void16-redux-mod-voronoi (Autodesk Fusion 360 design; units mm, degrees)
Autodesk Fusion 360 part; units mm, degrees
note: some values were not read from the file. Chosen so that the rebuilt part matches the saved one: which bodies a step acts on.
(part 1 of 2)
sketch "Sketch572" plane through (0, 0, 0) normal (0, 0, 1) x (1, 0, 0)
  line L0 (0, -3.5) -> (84.45, -3.5)
  line L1 (84.45, -3.5) -> (84.45, 110.5)
  line L2 (84.45, 110.5) -> (0, 110.5)
  line L3 (0, 110.5) -> (0, -3.5)
extrude "Extrude566" add sketch "Sketch572" along normal blind 28 makes body 1
sketch "Sketch573" plane through (0, 0, 0) normal (0, 0, 1) x (1, 0, 0)
  line L0 (0, -1.5) -> (0, -3.5)
  line L1 (0, -3.5) -> (2, -3.5)
  arc A0 (0, -1.5) -> (2, -3.5) centre (2, -1.5) ccw
  line L2 (82.45, -3.5) -> (84.45, -3.5)
  line L3 (84.45, -3.5) -> (84.45, -1.5)
  arc A1 (82.45, -3.5) -> (84.45, -1.5) centre (82.45, -1.5) ccw
  line L4 (0, 108.5) -> (0, 110.5)
  line L5 (0, 110.5) -> (2, 110.5)
  arc A2 (2, 110.5) -> (0, 108.5) centre (2, 108.5) ccw
  line L6 (84.45, 108.5) -> (84.45, 110.5)
  line L7 (84.45, 110.5) -> (82.45, 110.5)
  arc A3 (84.45, 108.5) -> (82.45, 110.5) centre (82.45, 108.5) ccw
extrude "Extrude567" cut sketch "Sketch573" along normal blind 29 from surface at -0.5 bodies 1
sketch "Sketch574" plane through (0, 0, 0) normal (0, 0, 1) x (1, 0, 0)
  line L0 (2.5, -1) -> (81.95, -1)
  line L1 (81.95, -1) -> (81.95, 108)
  line L2 (81.95, 108) -> (2.5, 108)
  line L3 (2.5, 108) -> (2.5, -1)
extrude "Extrude568" cut sketch "Sketch574" along normal blind 32 from surface at 3 bodies 1
sketch "Sketch575" plane through (0, 0, 0) normal (0, 0, 1) x (1, 0, 0)
  line L0 (0, -3.5) -> (9.5938, -3.5)
  line L1 (9.5938, -3.5) -> (9.1335, 3.9995)
  line L2 (9.1335, 3.9995) -> (0, 8.5442)
  line L3 (0, 8.5442) -> (0, -3.5)
  line L4 (12.0985, -3.5) -> (18.3911, -3.5)
  line L5 (18.3911, -3.5) -> (18.0613, 5.0352)
  line L6 (18.0613, 5.0352) -> (16.3047, 5.9151)
  line L7 (16.3047, 5.9151) -> (11.6393, 3.9832)
  line L8 (11.6393, 3.9832) -> (12.0985, -3.5)
  line L9 (28.2832, -3.5) -> (32.7635, -3.5)
  line L10 (32.7635, -3.5) -> (33.7632, 2.8558)
  line L11 (33.7632, 2.8558) -> (27.7947, 7.4257)
  line L12 (27.7947, 7.4257) -> (26.2488, 6.2436)
  line L13 (26.2488, 6.2436) -> (28.2832, -3.5)
  line L14 (35.2942, -3.5) -> (42.0807, -3.5)
  line L15 (42.0807, -3.5) -> (38.4125, 3.9707)
  line L16 (38.4125, 3.9707) -> (36.2593, 2.6358)
  line L17 (36.2593, 2.6358) -> (35.2942, -3.5)
  line L18 (47.3257, -3.5) -> (55.0973, -3.5)
  line L19 (55.0973, -3.5) -> (54.5198, 3.2184)
  line L20 (54.5198, 3.2184) -> (50.3743, 5.4144)
  line L21 (50.3743, 5.4144) -> (48.1848, 4.5961)
  line L22 (48.1848, 4.5961) -> (47.3257, -3.5)
  line L23 (65.7275, 0.3641) -> (66.0747, 4.2167)
  line L24 (66.0747, 4.2167) -> (62.9422, 6.9148)
  line L25 (62.9422, 6.9148) -> (58.4517, 4.1915)
  line L26 (58.4517, 4.1915) -> (65.7275, 0.3641)
  line L27 (67.9938, -3.5) -> (84.45, -3.5)
  line L28 (84.45, -3.5) -> (84.45, -1.6781)
  line L29 (84.45, -1.6781) -> (73.5187, 5.0876)
  line L30 (73.5187, 5.0876) -> (68.5438, 3.7617)
  line L31 (68.5438, 3.7617) -> (68.0524, -1.6911)
  line L32 (68.0524, -1.6911) -> (67.9938, -3.5)
  line L33 (17.4974, 14.9007) -> (17.5932, 8.0658)
  line L34 (17.5932, 8.0658) -> (19.4771, 7.1222)
  line L35 (19.4771, 7.1222) -> (24.3515, 7.94)
  line L36 (24.3515, 7.94) -> (26.628, 9.6807)
  line L37 (26.628, 9.6807) -> (27.2775, 14.3423)
  line L38 (27.2775, 14.3423) -> (22.9787, 16.94)
  line L39 (22.9787, 16.94) -> (17.4974, 14.9007)
  line L40 (29.7772, 14.1667) -> (29.1338, 9.549)
  line L41 (29.1338, 9.549) -> (35.1883, 4.9133)
  line L42 (35.1883, 4.9133) -> (38.1934, 6.7763)
  line L43 (38.1934, 6.7763) -> (39.7695, 8.0899)
  line L44 (39.7695, 8.0899) -> (38.6804, 13.743)
  line L45 (38.6804, 13.743) -> (33.0704, 15.838)
  line L46 (33.0704, 15.838) -> (29.7772, 14.1667)
  line L47 (41.1504, 14.1374) -> (42.229, 8.5388)
  line L48 (42.229, 8.5388) -> (47.0139, 6.8273)
  line L49 (47.0139, 6.8273) -> (49.3539, 7.7019)
  line L50 (49.3539, 7.7019) -> (50.5571, 14.6378)
  line L51 (50.5571, 14.6378) -> (45.7034, 17.5514)
  line L52 (45.7034, 17.5514) -> (41.1504, 14.1374)
  line L53 (64.1082, 13.4115) -> (64.2958, 9.0485)
  line L54 (64.2958, 9.0485) -> (67.693, 6.1222)
  line L55 (67.693, 6.1222) -> (72.5495, 7.4166)
  line L56 (72.5495, 7.4166) -> (73.0869, 13.5316)
  line L57 (73.0869, 13.5316) -> (68.6367, 15.9672)
  line L58 (68.6367, 15.9672) -> (64.1082, 13.4115)
  line L59 (84.45, 1.262) -> (84.45, 16.7844)
  line L60 (84.45, 16.7844) -> (75.5807, 13.3511)
  line L61 (75.5807, 13.3511) -> (75.0306, 7.092)
  line L62 (75.0306, 7.092) -> (84.45, 1.262)
  line L63 (0, 24.6419) -> (0, 13.7038)
  line L64 (0, 13.7038) -> (10.6487, 19.0743)
  line L65 (10.6487, 19.0743) -> (10.4802, 23.8257)
  line L66 (10.4802, 23.8257) -> (3.3627, 26.8204)
  line L67 (3.3627, 26.8204) -> (0, 24.6419)
  line L68 (12.9711, 24.1247) -> (13.1512, 19.0456)
  line L69 (13.1512, 19.0456) -> (16.3589, 17.1445)
  line L70 (16.3589, 17.1445) -> (21.7934, 19.1664)
  line L71 (21.7934, 19.1664) -> (21.4341, 24.0717)
  line L72 (21.4341, 24.0717) -> (15.5962, 26.4591)
  line L73 (15.5962, 26.4591) -> (12.9711, 24.1247)
  line L74 (23.914, 24.4368) -> (24.308, 19.0577)
  line L75 (24.308, 19.0577) -> (28.6821, 16.4145)
  line L76 (28.6821, 16.4145) -> (31.8341, 18.0142)
  line L77 (31.8341, 18.0142) -> (32.5774, 24.0793)
  line L78 (32.5774, 24.0793) -> (26.9027, 27.276)
  line L79 (26.9027, 27.276) -> (23.914, 24.4368)
  line L80 (35.0947, 24.0681) -> (34.3544, 18.0272)
  line L81 (34.3544, 18.0272) -> (39.5721, 16.0787)
  line L82 (39.5721, 16.0787) -> (44.3657, 19.6731)
  line L83 (44.3657, 19.6731) -> (44.3045, 23.3989)
  line L84 (44.3045, 23.3989) -> (39.1405, 27.0251)
  line L85 (39.1405, 27.0251) -> (35.0947, 24.0681)
  line L86 (46.8046, 23.4107) -> (46.8644, 19.7703)
  line L87 (46.8644, 19.7703) -> (52.0665, 16.6476)
  line L88 (52.0665, 16.6476) -> (56.5667, 18.2936)
  line L89 (56.5667, 18.2936) -> (56.6261, 23.5251)
  line L90 (56.6261, 23.5251) -> (50.9806, 26.3187)
  line L91 (50.9806, 26.3187) -> (46.8046, 23.4107)
  line L92 (59.1283, 23.7061) -> (59.0645, 18.0861)
  line L93 (59.0645, 18.0861) -> (62.8752, 15.5863)
  line L94 (62.8752, 15.5863) -> (67.4847, 18.1878)
  line L95 (67.4847, 18.1878) -> (68.5198, 24.8801)
  line L96 (68.5198, 24.8801) -> (62.8789, 26.8335)
  line L97 (62.8789, 26.8335) -> (59.1283, 23.7061)
  line L98 (84.45, 19.4652) -> (84.45, 21.1436)
  line L99 (84.45, 21.1436) -> (73.5373, 26.3106)
  line L100 (73.5373, 26.3106) -> (71.0566, 24.9259)
  line L101 (71.0566, 24.9259) -> (69.9967, 18.0728)
  line L102 (69.9967, 18.0728) -> (74.4942, 15.6113)
  line L103 (74.4942, 15.6113) -> (84.45, 19.4652)
  line L104 (4.7066, 28.9673) -> (11.4594, 26.1259)
  line L105 (11.4594, 26.1259) -> (14.1071, 28.4805)
  line L106 (14.1071, 28.4805) -> (14.1908, 33.5736)
  line L107 (14.1908, 33.5736) -> (9.2969, 36.221)
  line L108 (9.2969, 36.221) -> (6.0759, 34.5401)
  line L109 (6.0759, 34.5401) -> (4.7066, 28.9673)
  line L110 (16.6907, 33.5503) -> (16.6118, 28.7448)
  line L111 (16.6118, 28.7448) -> (22.3492, 26.3985)
  line L112 (22.3492, 26.3985) -> (25.4548, 29.3487)
  line L113 (25.4548, 29.3487) -> (25.3909, 34.4579)
  line L114 (25.3909, 34.4579) -> (22.5593, 36.6355)
  line L115 (22.5593, 36.6355) -> (16.6907, 33.5503)
  line L116 (27.8953, 34.1174) -> (27.9524, 29.5541)
  line L117 (27.9524, 29.5541) -> (33.8321, 26.2419)
  line L118 (33.8321, 26.2419) -> (37.8625, 29.1876)
  line L119 (37.8625, 29.1876) -> (37.7669, 33.732)
  line L120 (37.7669, 33.732) -> (34.4771, 35.8382)
  line L121 (34.4771, 35.8382) -> (27.8953, 34.1174)
  line L122 (40.2683, 33.6924) -> (40.3623, 29.222)
  line L123 (40.3623, 29.222) -> (45.5468, 25.5813)
  line L124 (45.5468, 25.5813) -> (49.6527, 28.4405)
  line L125 (49.6527, 28.4405) -> (49.9378, 34.5492)
  line L126 (49.9378, 34.5492) -> (45.9679, 36.8072)
  line L127 (45.9679, 36.8072) -> (40.2683, 33.6924)
  line L128 (52.4319, 34.3637) -> (52.1594, 28.5247)
  line L129 (52.1594, 28.5247) -> (57.7096, 25.7783)
  line L130 (57.7096, 25.7783) -> (61.2439, 28.7253)
  line L131 (61.2439, 28.7253) -> (60.3685, 32.9277)
  line L132 (60.3685, 32.9277) -> (55.7232, 35.5484)
  line L133 (55.7232, 35.5484) -> (52.4319, 34.3637)
  line L134 (62.8536, 33.2568) -> (63.6998, 29.1949)
  line L135 (63.6998, 29.1949) -> (69.7944, 27.0844)
  line L136 (69.7944, 27.0844) -> (72.2993, 28.4826)
  line L137 (72.2993, 28.4826) -> (72.7061, 33.4194)
  line L138 (72.7061, 33.4194) -> (67.6468, 37.2404)
  line L139 (67.6468, 37.2404) -> (62.8536, 33.2568)
  line L140 (84.45, 23.9097) -> (84.45, 40.4504)
  line L141 (84.45, 40.4504) -> (75.2087, 33.3483)
  line L142 (75.2087, 33.3483) -> (74.8071, 28.4754)
  line L143 (74.8071, 28.4754) -> (84.45, 23.9097)
  line L144 (2.1055, 41.2203) -> (4.9302, 36.9105)
  line L145 (4.9302, 36.9105) -> (5.0583, 36.829)
  line L146 (5.0583, 36.829) -> (8.1291, 38.4315)
  line L147 (8.1291, 38.4315) -> (8.7625, 44.9281)
  line L148 (8.7625, 44.9281) -> (5.114, 46.9429)
  line L149 (5.114, 46.9429) -> (3.1764, 45.3012)
  line L150 (3.1764, 45.3012) -> (2.1055, 41.2203)
  line L151 (11.2619, 44.8) -> (10.6321, 38.3411)
  line L152 (10.6321, 38.3411) -> (15.4615, 35.7285)
  line L153 (15.4615, 35.7285) -> (21.3912, 38.8458)
  line L154 (21.3912, 38.8458) -> (21.1586, 42.7915)
  line L155 (21.1586, 42.7915) -> (15.9886, 47.0495)
  line L156 (15.9886, 47.0495) -> (11.2619, 44.8)
  line L157 (23.6638, 42.778) -> (23.9007, 38.7577)
  line L158 (23.9007, 38.7577) -> (26.9097, 36.4437)
  line L159 (26.9097, 36.4437) -> (33.4266, 38.1475)
  line L160 (33.4266, 38.1475) -> (33.3406, 44.2394)
  line L161 (33.3406, 44.2394) -> (29.0152, 46.4456)
  line L162 (29.0152, 46.4456) -> (23.6638, 42.778)
  line L163 (35.8399, 44.3097) -> (35.9307, 37.876)
  line L164 (35.9307, 37.876) -> (39.0529, 35.8772)
  line L165 (39.0529, 35.8772) -> (44.7125, 38.9701)
  line L166 (44.7125, 38.9701) -> (44.5965, 43.8915)
  line L167 (44.5965, 43.8915) -> (40.3784, 47.0399)
  line L168 (40.3784, 47.0399) -> (35.8399, 44.3097)
  line L169 (47.0984, 43.8421) -> (47.213, 38.9751)
  line L170 (47.213, 38.9751) -> (51.3401, 36.6277)
  line L171 (51.3401, 36.6277) -> (54.7875, 37.8686)
  line L172 (54.7875, 37.8686) -> (56.2956, 43.9099)
  line L173 (56.2956, 43.9099) -> (51.1457, 46.3401)
  line L174 (51.1457, 46.3401) -> (47.0984, 43.8421)
  line L175 (58.8345, 43.7586) -> (57.282, 37.5394)
  line L176 (57.282, 37.5394) -> (61.3403, 35.2498)
  line L177 (61.3403, 35.2498) -> (66.3216, 39.3897)
  line L178 (66.3216, 39.3897) -> (66.088, 43.0389)
  line L179 (66.088, 43.0389) -> (62.1786, 45.5288)
  line L180 (62.1786, 45.5288) -> (58.8345, 43.7586)
  line L181 (5.9736, 49.3241) -> (10.1288, 47.0295)
  line L182 (10.1288, 47.0295) -> (15.0301, 49.362)
  line L183 (15.0301, 49.362) -> (15.6587, 53.6239)
  line L184 (15.6587, 53.6239) -> (11.3443, 57.7846)
  line L185 (11.3443, 57.7846) -> (4.5323, 53.1976)
  line L186 (4.5323, 53.1976) -> (5.9736, 49.3241)
  line L187 (18.1314, 53.2549) -> (17.5091, 49.0359)
  line L188 (17.5091, 49.0359) -> (22.4432, 44.9723)
  line L189 (22.4432, 44.9723) -> (27.6555, 48.5444)
  line L190 (27.6555, 48.5444) -> (27.5474, 53.0485)
  line L191 (27.5474, 53.0485) -> (21.7746, 55.1009)
  line L192 (21.7746, 55.1009) -> (18.1314, 53.2549)
  line L193 (30.0403, 53.3739) -> (30.1531, 48.6716)
  line L194 (30.1531, 48.6716) -> (34.5299, 46.4392)
  line L195 (34.5299, 46.4392) -> (39.1917, 49.2435)
  line L196 (39.1917, 49.2435) -> (39.1152, 53.9062)
  line L197 (39.1152, 53.9062) -> (33.237, 56.1053)
  line L198 (33.237, 56.1053) -> (30.0403, 53.3739)
  line L199 (41.611, 54.1823) -> (41.6931, 49.1782)
  line L200 (41.6931, 49.1782) -> (45.8985, 46.0393)
  line L201 (45.8985, 46.0393) -> (49.8653, 48.4877)
  line L202 (49.8653, 48.4877) -> (50.2706, 54.1099)
  line L203 (50.2706, 54.1099) -> (45.0819, 56.9347)
  line L204 (45.0819, 56.9347) -> (41.611, 54.1823)
  line L205 (52.765, 53.9424) -> (52.3745, 48.5247)
  line L206 (52.3745, 48.5247) -> (57.7247, 45.9998)
  line L207 (57.7247, 45.9998) -> (60.9835, 47.7249)
  line L208 (60.9835, 47.7249) -> (60.9612, 53.104)
  line L209 (60.9612, 53.104) -> (56.3989, 55.3457)
  line L210 (56.3989, 55.3457) -> (52.765, 53.9424)
  line L211 (63.4607, 53.2407) -> (63.4838, 47.6615)
  line L212 (63.4838, 47.6615) -> (67.3696, 45.1866)
  line L213 (67.3696, 45.1866) -> (73.5414, 48.2671)
  line L214 (73.5414, 48.2671) -> (72.5144, 54.1165)
  line L215 (72.5144, 54.1165) -> (68.4625, 56.7928)
  line L216 (68.4625, 56.7928) -> (63.4607, 53.2407)
  line L217 (84.45, 43.7394) -> (84.45, 58.9147)
  line L218 (84.45, 58.9147) -> (75.0441, 54.1652)
  line L219 (75.0441, 54.1652) -> (76.0615, 48.3703)
  line L220 (76.0615, 48.3703) -> (84.45, 43.7394)
  line L221 (0, 69.0808) -> (0, 56.6662)
  line L222 (0, 56.6662) -> (2.9358, 55.1366)
  line L223 (2.9358, 55.1366) -> (10.1876, 60.0197)
  line L224 (10.1876, 60.0197) -> (9.914, 63.973)
  line L225 (9.914, 63.973) -> (1.8674, 69.0503)
  line L226 (1.8674, 69.0503) -> (0, 69.0808)
  line L227 (12.4205, 63.9653) -> (12.6983, 59.952)
  line L228 (12.6983, 59.952) -> (17.2171, 55.5942)
  line L229 (17.2171, 55.5942) -> (20.5627, 57.2894)
  line L230 (20.5627, 57.2894) -> (21.8412, 64.719)
  line L231 (21.8412, 64.719) -> (16.3821, 66.0508)
  line L232 (16.3821, 66.0508) -> (12.4205, 63.9653)
  line L233 (24.3951, 64.8189) -> (23.0984, 57.2836)
  line L234 (23.0984, 57.2836) -> (28.514, 55.3581)
  line L235 (28.514, 55.3581) -> (31.6396, 58.0287)
  line L236 (31.6396, 58.0287) -> (30.6879, 63.9531)
  line L237 (30.6879, 63.9531) -> (27.2484, 66.233)
  line L238 (27.2484, 66.233) -> (24.3951, 64.8189)
  line L239 (33.2272, 63.9078) -> (34.104, 58.4502)
  line L240 (34.104, 58.4502) -> (40.1276, 56.1966)
  line L241 (40.1276, 56.1966) -> (43.7319, 59.0548)
  line L242 (43.7319, 59.0548) -> (43.9492, 63.5829)
  line L243 (43.9492, 63.5829) -> (39.4165, 66.4165)
  line L244 (39.4165, 66.4165) -> (33.2272, 63.9078)
  line L245 (46.452, 63.5807) -> (46.2394, 59.1511)
  line L246 (46.2394, 59.1511) -> (51.6647, 56.1974)
  line L247 (51.6647, 56.1974) -> (55.2211, 57.5708)
  line L248 (55.2211, 57.5708) -> (55.3137, 64.1101)
  line L249 (55.3137, 64.1101) -> (49.9567, 66.0238)
  line L250 (49.9567, 66.0238) -> (46.452, 63.5807)
  line L251 (57.8158, 64.2432) -> (57.7201, 57.482)
  line L252 (57.7201, 57.482) -> (62.0912, 55.3343)
  line L253 (62.0912, 55.3343) -> (67.1656, 58.9382)
  line L254 (67.1656, 58.9382) -> (67.0042, 63.8929)
  line L255 (67.0042, 63.8929) -> (62.2691, 66.7036)
  line L256 (62.2691, 66.7036) -> (57.8158, 64.2432)
  line L257 (84.45, 61.7153) -> (84.45, 63.8136)
  line L258 (84.45, 63.8136) -> (77.4052, 69.187)
  line L259 (77.4052, 69.187) -> (69.5033, 63.9609)
  line L260 (69.5033, 63.9609) -> (69.6651, 58.9946)
  line L261 (69.6651, 58.9946) -> (73.7363, 56.3055)
  line L262 (73.7363, 56.3055) -> (84.45, 61.7153)
  line L263 (4.2762, 70.4864) -> (11.1737, 66.1342)
  line L264 (11.1737, 66.1342) -> (15.008, 68.1527)
  line L265 (15.008, 68.1527) -> (15.4108, 75.727)
  line L266 (15.4108, 75.727) -> (11.9553, 77.6511)
  line L267 (11.9553, 77.6511) -> (4.2762, 70.4864)
  line L268 (17.9008, 75.4729) -> (17.5218, 68.3461)
  line L269 (17.5218, 68.3461) -> (23.1243, 66.9793)
  line L270 (23.1243, 66.9793) -> (26.1217, 68.4648)
  line L271 (26.1217, 68.4648) -> (26.3453, 73.6548)
  line L272 (26.3453, 73.6548) -> (22.046, 76.6112)
  line L273 (22.046, 76.6112) -> (17.9008, 75.4729)
  line L274 (28.8457, 73.6109) -> (28.6179, 68.3246)
  line L275 (28.6179, 68.3246) -> (31.9764, 66.0984)
  line L276 (31.9764, 66.0984) -> (38.2604, 68.6454)
  line L277 (38.2604, 68.6454) -> (38.0989, 73.5822)
  line L278 (38.0989, 73.5822) -> (33.2869, 76.6232)
  line L279 (33.2869, 76.6232) -> (28.8457, 73.6109)
  line L280 (40.6009, 73.5622) -> (40.7658, 68.5213)
  line L281 (40.7658, 68.5213) -> (45.1954, 65.7522)
  line L282 (45.1954, 65.7522) -> (48.5589, 68.0969)
  line L283 (48.5589, 68.0969) -> (48.9328, 74.3327)
  line L284 (48.9328, 74.3327) -> (46.0081, 76.5598)
  line L285 (46.0081, 76.5598) -> (40.6009, 73.5622)
  line L286 (51.4188, 74.0232) -> (51.0743, 68.2793)
  line L287 (51.0743, 68.2793) -> (56.4655, 66.3533)
  line L288 (56.4655, 66.3533) -> (60.9407, 68.8258)
  line L289 (60.9407, 68.8258) -> (60.267, 73.9347)
  line L290 (60.267, 73.9347) -> (57.3848, 76.1484)
  line L291 (57.3848, 76.1484) -> (51.4188, 74.0232)
  line L292 (67.6869, 76.6064) -> (62.7898, 73.9255)
  line L293 (62.7898, 73.9255) -> (63.4514, 68.9091)
  line L294 (63.4514, 68.9091) -> (68.1953, 66.0931)
  line L295 (68.1953, 66.0931) -> (76.1164, 71.3319)
  line L296 (76.1164, 71.3319) -> (76.0166, 72.0979)
  line L297 (76.0166, 72.0979) -> (67.6869, 76.6064)
  line L298 (0, 83.0517) -> (0, 71.5812)
  line L299 (0, 71.5812) -> (1.7542, 71.5525)
  line L300 (1.7542, 71.5525) -> (10.4214, 79.6391)
  line L301 (10.4214, 79.6391) -> (9.7366, 83.6036)
  line L302 (9.7366, 83.6036) -> (0, 83.0517)
  line L303 (24.0822, 85.0868) -> (23.5774, 78.5921)
  line L304 (23.5774, 78.5921) -> (27.6288, 75.8063)
  line L305 (27.6288, 75.8063) -> (32.0923, 78.8337)
  line L306 (32.0923, 78.8337) -> (32.5475, 82.4904)
  line L307 (32.5475, 82.4904) -> (27.2658, 86.2587)
  line L308 (27.2658, 86.2587) -> (24.0822, 85.0868)
  line L309 (35.0515, 82.3674) -> (34.6012, 78.75)
  line L310 (34.6012, 78.75) -> (39.3682, 75.7373)
  line L311 (39.3682, 75.7373) -> (44.7879, 78.7418)
  line L312 (44.7879, 78.7418) -> (44.2103, 84.3411)
  line L313 (44.2103, 84.3411) -> (40.62, 86.2398)
  line L314 (40.62, 86.2398) -> (35.0515, 82.3674)
  line L315 (46.719, 84.3856) -> (47.3038, 78.7154)
  line L316 (47.3038, 78.7154) -> (50.439, 76.3281)
  line L317 (50.439, 76.3281) -> (56.3587, 78.4368)
  line L318 (56.3587, 78.4368) -> (56.3723, 83.8601)
  line L319 (56.3723, 83.8601) -> (50.2849, 86.089)
  line L320 (50.2849, 86.089) -> (46.719, 84.3856)
  line L321 (58.8729, 84.1362) -> (58.858, 78.1692)
  line L322 (58.858, 78.1692) -> (61.5535, 76.0988)
  line L323 (61.5535, 76.0988) -> (66.4865, 78.7994)
  line L324 (66.4865, 78.7994) -> (66.9203, 84.7231)
  line L325 (66.9203, 84.7231) -> (61.692, 86.424)
  line L326 (61.692, 86.424) -> (58.8729, 84.1362)
  line L327 (72.5997, 86.3423) -> (69.4326, 84.7999)
  line L328 (69.4326, 84.7999) -> (68.9892, 78.7442)
  line L329 (68.9892, 78.7442) -> (76.5476, 74.6532)
  line L330 (76.5476, 74.6532) -> (78.9962, 80.5865)
  line L331 (78.9962, 80.5865) -> (72.5997, 86.3423)
  line L332 (11.1555, 87.0697) -> (15.0434, 90.3681)
  line L333 (15.0434, 90.3681) -> (15.1256, 94.124)
  line L334 (15.1256, 94.124) -> (10.5379, 97.1905)
  line L335 (10.5379, 97.1905) -> (5.4734, 94.7053)
  line L336 (5.4734, 94.7053) -> (11.1555, 87.0697)
  line L337 (31.4995, 98.4229) -> (28.8774, 88.1799)
  line L338 (28.8774, 88.1799) -> (33.8892, 84.6042)
  line L339 (33.8892, 84.6042) -> (39.1354, 88.2525)
  line L340 (39.1354, 88.2525) -> (37.0101, 98.2076)
  line L341 (37.0101, 98.2076) -> (31.6021, 98.4443)
  line L342 (31.6021, 98.4443) -> (31.4995, 98.4229)
  line L343 (39.4217, 98.8856) -> (41.6319, 88.5327)
  line L344 (41.6319, 88.5327) -> (45.4137, 86.5327)
  line L345 (45.4137, 86.5327) -> (49.0932, 88.2904)
  line L346 (49.0932, 88.2904) -> (50.0863, 94.3257)
  line L347 (50.0863, 94.3257) -> (39.6425, 99.048)
  line L348 (39.6425, 99.048) -> (39.4217, 98.8856)
  line L349 (52.6124, 94.2799) -> (51.6221, 88.2617)
  line L350 (51.6221, 88.2617) -> (57.3878, 86.1506)
  line L351 (57.3878, 86.1506) -> (60.1357, 88.3807)
  line L352 (60.1357, 88.3807) -> (59.6428, 94.8014)
  line L353 (59.6428, 94.8014) -> (57.1386, 96.8701)
  line L354 (57.1386, 96.8701) -> (52.6124, 94.2799)
  line L355 (62.1726, 94.5094) -> (62.6145, 88.7529)
  line L356 (62.6145, 88.7529) -> (68.1451, 86.9536)
  line L357 (68.1451, 86.9536) -> (71.7234, 88.6962)
  line L358 (71.7234, 88.6962) -> (72.7403, 93.178)
  line L359 (72.7403, 93.178) -> (68.5318, 96.3546)
  line L360 (68.5318, 96.3546) -> (62.1726, 94.5094)
  line L361 (84.45, 88.1142) -> (84.45, 98.4831)
  line L362 (84.45, 98.4831) -> (76.4474, 93.6273)
  line L363 (76.4474, 93.6273) -> (84.45, 88.1142)
  line L364 (8.2463, 110.5) -> (0, 110.5)
  line L365 (0, 110.5) -> (0, 96.5387)
  line L366 (0, 96.5387) -> (3.3033, 96.4252)
  line L367 (3.3033, 96.4252) -> (9.3074, 99.3715)
  line L368 (9.3074, 99.3715) -> (8.2463, 110.5)
  line L369 (14.1848, 110.5) -> (10.7576, 110.5)
  line L370 (10.7576, 110.5) -> (11.8218, 99.3394)
  line L371 (11.8218, 99.3394) -> (16.3415, 96.3183)
  line L372 (16.3415, 96.3183) -> (16.7779, 96.6519)
  line L373 (16.7779, 96.6519) -> (16.4734, 107.8826)
  line L374 (16.4734, 107.8826) -> (14.1848, 110.5)
  line L375 (54.5213, 110.5) -> (46.5468, 110.5)
  line L376 (46.5468, 110.5) -> (41.2486, 101.0655)
  line L377 (41.2486, 101.0655) -> (51.4088, 96.4715)
  line L378 (51.4088, 96.4715) -> (55.961, 99.0767)
  line L379 (55.961, 99.0767) -> (55.8021, 101.1391)
  line L380 (55.8021, 101.1391) -> (54.5213, 110.5)
  line L381 (58.3855, 100.1523) -> (58.4736, 99.01)
  line L382 (58.4736, 99.01) -> (61.135, 96.8114)
  line L383 (61.135, 96.8114) -> (67.5752, 98.6801)
  line L384 (67.5752, 98.6801) -> (67.6807, 101.1012)
  line L385 (67.6807, 101.1012) -> (58.3855, 100.1523)
extrude "Extrude569" add sketch "Sketch575" along normal blind 36 from surface at -6 separate body makes body 2 at (44.6353, 99.5341, 6) makes body 3 at (0, 105.8462, 6) makes body 4 at (66.4121, 95.7395, 6) makes body 5 at (46.605, 95.8998, 6) makes body 6 at (7.3674, 92.1601, 6) makes body 7 at (58.868, 82.1472, 6) makes body 8 at (38.7639, 84.949, 18) makes body 9 at (4.6433, 74.248, 6) makes body 10 at (55.3961, 75.44, 6) makes body 11 at (36.1657, 67.7964, 18) makes body 12 at (9.3956, 75.2629, 18) makes body 13 at (57.7839, 61.9895, 18) makes body 14 at (37.3534, 65.5803, 6) makes body 15 at (20.9888, 59.766, 18) makes body 16 at (84.45, 48.7978, 6) makes body 17 at (54.1579, 47.6831, 6) makes body 18 at (37.1558, 54.6392, 6) makes body 19 at (19.1538, 47.6814, 6) makes body 20 at (63.0007, 36.6298, 6) makes body 21 at (40.9394, 36.9081, 6) makes body 22 at (17.438, 36.7676, 6) makes body 23 at (84.45, 29.4232, 6) makes body 24 at (54.0095, 27.6092, 6) makes body 25 at (32.2832, 35.2646, 18) makes body 26 at (6.9575, 28.0202, 6) makes body 27 at (67.8298, 20.4186, 6) makes body 28 at (42.5831, 24.6076, 6) makes body 29 at (19.4881, 24.8675, 6) makes body 30 at (84.45, 6.4361, 6) makes body 31 at (49.7549, 10.0139, 18) makes body 32 at (17.5294, 12.6224, 18) makes body 33 at (60.877, 2.9157, 6) makes body 34 at (40.858, -1.0098, 6) makes body 35 at (18.2812, -0.6549, 6) makes body 36 at (26.9269, 2.9957, 6) makes body 37 at (47.8984, 1.8974, 18) makes body 38 at (73.4792, -3.5, 6) makes body 39 at (31.152, 8.0038, 6) makes body 40 at (72.7286, 9.4549, 18) makes body 41 at (3.5496, 15.494, 6) makes body 42 at (30.6858, 25.1449, 6) makes body 43 at (54.7442, 24.4563, 6) makes body 44 at (80.8124, 22.8659, 6) makes body 45 at (20.6031, 35.6071, 6) makes body 46 at (44.068, 35.7689, 6) makes body 47 at (65.7313, 28.4914, 6) makes body 48 at (8.3402, 40.597, 6) makes body 49 at (29.082, 37.0116, 18) makes body 50 at (55.2902, 39.8824, 6) makes body 51 at (9.0737, 56.2556, 6) makes body 52 at (0, 4.5295, 6) makes body 53 at (48.541, 55.0515, 18) makes body 54 at (69.4269, 46.2134, 18) makes body 55 at (0, 64.9426, 6) makes body 56 at (23.9629, 62.3071, 6) makes body 57 at (55.252, 59.7506, 6) makes body 58 at (77.3075, 58.1088, 18) makes body 59 at (17.7745, 73.0973, 6) makes body 60 at (48.6836, 70.1755, 6) makes body 61 at (70.8357, 67.8394, 6) makes body 62 at (23.9139, 82.9219, 6) makes body 63 at (54.3431, 84.6031, 6) makes body 64 at (76.864, 82.5051, 18) makes body 65 at (30.6254, 95.0086, 6) makes body 66 at (59.9714, 90.5209, 6) makes body 67 at (84.45, 91.5705, 6) makes body 68 at (16.6764, 100.3955, 6) makes body 69 at (64.5823, 100.7849, 18)
move_body "Move584" bodies 2 to x (0.991592, 0.008841, 0.129102) y (0.008841, 0.990703, -0.135753) z (-0.129102, 0.135753, 0.982295) at (1.043, -1.0967, 7.986)
move_body "Move585" bodies 3 to x (0.995047, 0.007992, -0.099087) y (0.007992, 0.987106, 0.159865) z (0.099087, -0.159865, 0.982153) at (-1.9928, 3.2152, -15.8648)
move_body "Move586" bodies 4 to x (0.994433, 0.011641, 0.104726) y (0.011641, 0.975656, -0.218996) z (-0.104726, 0.218996, 0.970089) at (0.5653, -1.182, 13.3664)
move_body "Move587" bodies 5 to x (0.988041, -0.017698, -0.153174) y (-0.017698, 0.97381, -0.226673) z (0.153174, 0.226673, 0.961851) at (0.3393, 0.5021, 28.346)
move_body "Move588" bodies 6 to x (0.968969, 0.002343, 0.247172) y (0.002343, 0.999823, -0.018664) z (-0.247172, 0.018664, 0.968792) at (3.0698, -0.2318, -0.4517)
move_body "Move589" bodies 7 to x (0.977564, 0.020464, -0.209644) y (0.020464, 0.981335, 0.191215) z (0.209644, -0.191215, 0.958898) at (-2.7677, 2.5244, -1.8608)
move_body "Move590" bodies 8 to x (0.998968, -0.005949, -0.045022) y (-0.005949, 0.965695, -0.25961) z (0.045022, 0.25961, 0.964663) at (-0.0175, -0.1009, 23.2366)
move_body "Move591" bodies 9 to x (0.987423, 0.004942, 0.158025) y (0.004942, 0.998058, -0.062096) z (-0.158025, 0.062096, 0.985481) at (1.5784, -0.6202, 4.1681)
move_body "Move592" bodies 10 to x (0.99475, -0.01008, -0.101838) y (-0.01008, 0.980646, -0.195532) z (0.101838, 0.195532, 0.975395) at (-0.2098, -0.4028, 19.9308)
move_body "Move593" bodies 11 to x (0.966183, 0.017671, -0.257253) y (0.017671, 0.990766, 0.134424) z (0.257253, -0.134424, 0.956949) at (-3.2172, 1.6811, -0.4737)
move_body "Move594" bodies 12 to x (0.993128, -0.009793, -0.116619) y (-0.009793, 0.986043, -0.166201) z (0.116619, 0.166201, 0.979172) at (-0.6277, -0.8946, 13.3465)
move_body "Move595" bodies 13 to x (0.983187, 0.000142, 0.182601) y (0.000142, 0.999999, -0.001542) z (-0.182601, 0.001542, 0.983186) at (3.2324, -0.0273, -11.1063)
move_body "Move596" bodies 14 to x (0.995747, -0.007957, 0.091783) y (-0.007957, 0.985112, 0.171731) z (-0.091783, -0.171731, 0.980859) at (1.7533, 3.2806, -13.8403)
move_body "Move597" bodies 15 to x (0.994867, -0.009808, 0.100713) y (-0.009808, 0.981258, 0.192447) z (-0.100713, -0.192447, 0.976126) at (1.893, 3.6173, -13.1439)
move_body "Move598" bodies 16 to x (0.9987, 0.003972, 0.050813) y (0.003972, 0.987858, -0.155306) z (-0.050813, 0.155306, 0.986559) at (0.5095, -1.5573, 4.0805)
move_body "Move599" bodies 17 to x (0.968799, -0.018725, 0.247139) y (-0.018725, 0.988762, 0.148319) z (-0.247139, -0.148319, 0.957561) at (5.6829, 3.4106, -21.0141)
move_body "Move600" bodies 18 to x (0.989264, -0.007666, -0.145936) y (-0.007666, 0.994525, -0.104213) z (0.145936, 0.104213, 0.98379) at (-0.9865, -0.7045, 10.5895)
move_body "Move601" bodies 19 to x (0.978538, 0.004975, 0.206004) y (0.004975, 0.998847, -0.047753) z (-0.206004, 0.047753, 0.977385) at (2.7078, -0.6277, -1.9913)
move_body "Move602" bodies 20 to x (0.979527, -0.021522, 0.200161) y (-0.021522, 0.977376, 0.210412) z (-0.200161, -0.210412, 0.956902) at (4.5365, 4.7688, -20.3515)
move_body "Move603" bodies 21 to x (0.976858, -0.005031, -0.213831) y (-0.005031, 0.998906, -0.046487) z (0.213831, 0.046487, 0.975764) at (-1.4253, -0.3099, 10.8304)
move_body "Move604" bodies 22 to x (0.996945, -0.011117, 0.07731) y (-0.011117, 0.959546, 0.281331) z (-0.07731, -0.281331, 0.956491) at (1.4367, 5.2283, -12.3598)
move_body "Move605" bodies 23 to x (0.984696, 0.003078, -0.174254) y (0.003078, 0.999381, 0.03505) z (0.174254, -0.03505, 0.984077) at (-0.9715, 0.1954, 12.9387)
move_body "Move606" bodies 24 to x (0.998925, -0.005398, 0.046044) y (-0.005398, 0.972899, 0.231169) z (-0.046044, -0.231169, 0.971824) at (0.779, 3.9111, -9.361)
move_body "Move607" bodies 25 to x (0.98641, 0.000173, 0.1643) y (0.000173, 0.999998, -0.00209) z (-0.1643, 0.00209, 0.986408) at (2.413, -0.0307, -5.174)
move_body "Move608" bodies 26 to x (0.999988, 0.000678, -0.004883) y (0.000678, 0.962127, 0.272602) z (0.004883, -0.272602, 0.962115) at (-0.0796, 4.4455, -7.9972)
move_body "Move609" bodies 27 to x (0.99916, -0.003341, -0.040854) y (-0.003341, 0.986717, -0.162413) z (0.040854, 0.162413, 0.985877) at (-0.3658, -1.4541, 6.2204)
move_body "Move610" bodies 28 to x (0.990065, 0.014611, -0.139846) y (0.014611, 0.97851, 0.20568) z (0.139846, -0.20568, 0.968576) at (-1.602, 2.3562, 1.4487)
move_body "Move611" bodies 29 to x (0.981598, 0.019624, 0.189947) y (0.019624, 0.979073, -0.202562) z (-0.189947, 0.202562, 0.960671) at (2.1714, -2.3156, 1.5865)
move_body "Move612" bodies 30 to x (0.990758, 0.013688, -0.134949) y (0.013688, 0.979727, 0.199868) z (0.134949, -0.199868, 0.970485) at (-1.0059, 1.4899, 9.3116)
move_body "Move613" bodies 31 to x (0.993364, 0.011438, 0.114445) y (0.011438, 0.980286, -0.197253) z (-0.114445, 0.197253, 0.97365) at (1.5382, -2.6512, -2.5271)
move_body "Move614" bodies 32 to x (0.969777, 0.008933, 0.243828) y (0.008933, 0.997359, -0.072071) z (-0.243828, 0.072071, 0.967137) at (3.4951, -1.0331, -4.1972)
move_body "Move615" bodies 33 to x (0.988391, -0.01512, 0.151179) y (-0.01512, 0.980307, 0.196899) z (-0.151179, -0.196899, 0.968698) at (2.592, 3.3759, -9.7539)
move_body "Move616" bodies 34 to x (0.971429, -0.012616, 0.236996) y (-0.012616, 0.99443, 0.104645) z (-0.236996, -0.104645, 0.965858) at (3.9523, 1.7451, -8.7837)
move_body "Move617" bodies 35 to x (0.997071, -0.010919, -0.075703) y (-0.010919, 0.959297, -0.282187) z (0.075703, 0.282187, 0.956368) at (-0.8513, -3.1731, 2.001)
move_body "Move618" bodies 36 to x (0.996566, 0.006927, 0.082518) y (0.006927, 0.98603, -0.166422) z (-0.082518, 0.166422, 0.982596) at (1.0797, -2.1775, -1.9405)
move_body "Move619" bodies 37 to x (0.99354, -0.01449, 0.112549) y (-0.01449, 0.967495, 0.252474) z (-0.112549, -0.252474, 0.961036) at (1.6953, 3.8029, -5.5379)
move_body "Move620" bodies 38 to x (0.991452, -0.007979, -0.130227) y (-0.007979, 0.992551, -0.121565) z (0.130227, 0.121565, 0.984003) at (-0.9049, -0.8447, 10.2146)
move_body "Move621" bodies 39 to x (0.973167, 0.008063, 0.229958) y (0.008063, 0.997577, -0.069103) z (-0.229958, 0.069103, 0.970744) at (3.6003, -1.0819, -6.8544)
move_body "Move622" bodies 40 to x (0.991536, 0.005832, 0.129704) y (0.005832, 0.995981, -0.089372) z (-0.129704, 0.089372, 0.987517) at (2.0727, -1.4282, -7.7605)
move_body "Move623" bodies 41 to x (0.971876, -0.009017, -0.235321) y (-0.009017, 0.997109, -0.075446) z (0.235321, 0.075446, 0.968985) at (-2.4914, -0.7988, 3.1538)
move_body "Move624" bodies 42 to x (0.991648, 0.00743, 0.128759) y (0.00743, 0.993391, -0.11454) z (-0.128759, 0.11454, 0.985039) at (1.6187, -1.44, -0.9552)
move_body "Move625" bodies 43 to x (0.997956, 0.005882, 0.063632) y (0.005882, 0.983071, -0.183131) z (-0.063632, 0.183131, 0.981027) at (0.7429, -2.1381, 0.8712)
move_body "Move626" bodies 44 to x (0.983544, 0.003396, 0.180639) y (0.003396, 0.999299, -0.037276) z (-0.180639, 0.037276, 0.982843) at (3.3673, -0.6949, -12.9623)
move_body "Move627" bodies 45 to x (0.974924, -0.002209, -0.222529) y (-0.002209, 0.999805, -0.019603) z (0.222529, 0.019603, 0.974729) at (-2.0733, -0.1826, 5.6016)
move_body "Move628" bodies 46 to x (0.990236, -0.006735, -0.139238) y (-0.006735, 0.995354, -0.096044) z (0.139238, 0.096044, 0.98559) at (-1.0204, -0.7038, 9.449)
move_body "Move629" bodies 47 to x (0.987956, -0.002038, -0.154724) y (-0.002038, 0.999655, -0.026183) z (0.154724, 0.026183, 0.987611) at (-0.9748, -0.165, 11.4779)
move_body "Move630" bodies 48 to x (0.989236, 0.009238, 0.146034) y (0.009238, 0.992071, -0.12534) z (-0.146034, 0.12534, 0.981307) at (1.4239, -1.2222, 4.6807)
move_body "Move631" bodies 49 to x (0.997617, 0.007078, -0.068626) y (0.007078, 0.978974, 0.203861) z (0.068626, -0.203861, 0.976592) at (-1.0488, 3.1157, -6.2091)
move_body "Move632" bodies 50 to x (0.991903, 0.015832, -0.126008) y (0.015832, 0.969046, 0.246371) z (0.126008, -0.246371, 0.960949) at (-1.7503, 3.4221, -3.2376)
move_body "Move633" bodies 51 to x (0.99703, 0.010082, 0.076348) y (0.010082, 0.965771, -0.2592) z (-0.076348, 0.2592, 0.962801) at (0.4178, -1.4183, 13.2595)
move_body "Move634" bodies 52 to x (0.990192, 0.007307, 0.139521) y (0.007307, 0.994556, -0.103944) z (-0.139521, 0.103944, 0.984748) at (1.7029, -1.2686, -0.2241)
move_body "Move635" bodies 53 to x (0.987427, -0.017075, 0.157152) y (-0.017075, 0.976812, 0.213416) z (-0.157152, -0.213416, 0.964239) at (3.3426, 4.5393, -17.7787)
move_body "Move636" bodies 54 to x (0.993903, -0.008274, -0.109947) y (-0.008274, 0.988773, -0.149199) z (0.109947, 0.149199, 0.982676) at (-0.4798, -0.6511, 15.347)
move_body "Move637" bodies 55 to x (0.987258, 0.016905, -0.158225) y (0.016905, 0.977571, 0.209928) z (0.158225, -0.209928, 0.964829) at (-2.8838, 3.8261, -11.8104)
move_body "Move638" bodies 56 to x (0.990899, -0.013645, 0.133917) y (-0.013645, 0.979544, 0.200769) z (-0.133917, -0.200769, 0.970442) at (2.6857, 4.0263, -15.5164)
move_body "Move639" bodies 57 to x (0.993027, -0.014789, 0.116952) y (-0.014789, 0.968633, 0.248054) z (-0.116952, -0.248054, 0.961661) at (2.6612, 5.6444, -20.6371)
move_body "Move640" bodies 58 to x (0.966428, -0.013481, -0.256585) y (-0.013481, 0.994587, -0.103031) z (0.256585, 0.103031, 0.961014) at (0.3511, 0.141, 26.6837)
move_body "Move641" bodies 59 to x (0.97952, 0.001733, 0.201341) y (0.001733, 0.999853, -0.017037) z (-0.201341, 0.017037, 0.979373) at (2.7409, -0.2319, -2.9454)
move_body "Move642" bodies 60 to x (0.965663, -0.011692, 0.259535) y (-0.011692, 0.996019, 0.088376) z (-0.259535, -0.088376, 0.961681) at (5.4836, 1.8673, -17.4472)
move_body "Move643" bodies 61 to x (0.964956, -0.003714, 0.262387) y (-0.003714, 0.999606, 0.02781) z (-0.262387, -0.02781, 0.964562) at (5.8476, 0.6198, -19.7825)
move_body "Move644" bodies 62 to x (0.980267, -0.019043, -0.196759) y (-0.019043, 0.981624, -0.189875) z (0.196759, 0.189875, 0.961891) at (-0.2643, -0.255, 21.3649)
move_body "Move645" bodies 63 to x (0.979629, -0.009057, -0.200611) y (-0.009057, 0.995973, -0.089197) z (0.200611, 0.089197, 0.975602) at (-0.6218, -0.2765, 17.8769)
move_body "Move646" bodies 64 to x (0.983624, -0.004796, -0.180169) y (-0.004796, 0.998595, -0.052768) z (0.180169, 0.052768, 0.982219) at (-0.5642, -0.1653, 17.7923)
move_body "Move647" bodies 65 to x (0.981994, 0.006723, -0.188795) y (0.006723, 0.99749, 0.070487) z (0.188795, -0.070487, 0.979484) at (-2.2685, 0.847, 0.2151)
move_body "Move648" bodies 66 to x (0.999183, -0.003871, 0.040235) y (-0.003871, 0.98166, 0.190599) z (-0.040235, -0.190599, 0.980843) at (0.8828, 4.1818, -19.4602)
move_body "Move649" bodies 67 to x (0.985086, -0.020441, -0.170845) y (-0.020441, 0.971985, -0.234152) z (0.170845, 0.234152, 0.957071) at (1.0568, 1.4483, 36.1055)
move_body "Move650" bodies 68 to x (0.997923, -0.005172, 0.064202) y (-0.005172, 0.987118, 0.159913) z (-0.064202, -0.159913, 0.985041) at (1.3339, 3.3223, -17.2409)
move_body "Move651" bodies 69 to x (0.965762, 0.016489, 0.258904) y (0.016489, 0.992059, -0.124689) z (-0.258904, 0.124689, 0.957821) at (3.6333, -1.7498, -3.4746)
combine "Combine170" operation cut target body 1 tool bodies 2 3 4 5 6 7 8 9 10 11 12 13 14 15 16 17 18 19 20 21 22 23 24 25 26 27 28 29 30 31 32 33 34 35 36 37 38 39 40 41 42 43 44 45 46 47 48 49 50 51 52 53 54 55 56 57 58 59 60 61 62 63 64 65 66 67 68 69
sketch "Sketch576" plane through (0, 0, 0) normal (0, 0, 1) x (1, 0, 0)
  circle A0 centre (20, 102.4) radius 3.5
  circle A1 centre (64, 102.4) radius 3.5
  circle A2 centre (4.5, 89) radius 3.5
  circle A3 centre (79.95, 89) radius 3.5
extrude "Extrude570" add sketch "Sketch576" along normal blind 30 separate body makes body 70 at (7.7252, 87.6405, 20) makes body 71 at (67.0738, 100.7261, 20) makes body 72 at (23.0738, 104.0739, 20) makes body 73 at (78.8353, 85.6823, 10)
combine "Combine171" operation add target body 1 tool bodies 70 71 72 73
sketch "Sketch577" plane through (0, 0, 0) normal (0, 0, 1) x (1, 0, 0)
  circle A0 centre (23.175, 0.9) radius 3.25
  circle A1 centre (42.225, 0.9) radius 3.25
  circle A2 centre (61.275, 0.9) radius 3.25
extrude "Extrude571" add sketch "Sketch577" along normal blind 30 separate body makes body 74 at (26.4089, 0.5764, 20) makes body 75 at (45.4589, 0.5764, 20) makes body 76 at (64.5089, 0.5764, 20)
combine "Combine172" operation add target body 1 tool bodies 74 75 76
sketch "Sketch578" plane through (0, 0, 0) normal (0, 0, 1) x (1, 0, 0)
  line L0 (19, 67.7) -> (21, 67.7)
  line L1 (21, 67.7) -> (21, 108.5)
  line L2 (21, 108.5) -> (19, 108.5)
  line L3 (19, 108.5) -> (19, 67.7)
  line L4 (39, 67.7) -> (41, 67.7)
  line L5 (41, 67.7) -> (41, 108.5)
  line L6 (41, 108.5) -> (39, 108.5)
  line L7 (39, 108.5) -> (39, 67.7)
extrude "Extrude572" add sketch "Sketch578" along normal blind 4.5 separate body makes body 77 at (19, 94.9, 1.5) makes body 78 at (39, 94.9, 1.5)
combine "Combine173" operation add target body 1 tool bodies 77 78
sketch "Sketch579" plane through (0, 0, 0) normal (0, 0, 1) x (1, 0, 0)
  line L0 (21, 67.7) -> (39, 67.7)
  line L1 (39, 67.7) -> (39, 108.5)
  line L2 (39, 108.5) -> (21, 108.5)
  line L3 (21, 108.5) -> (21, 67.7)
extrude "Extrude573" add sketch "Sketch579" along normal blind 4.5 separate body makes body 79
combine "Combine174" operation add target body 1 tool bodies 79
sketch "Sketch580" plane through (0, 0, 0) normal (0, 0, 1) x (1, 0, 0)
  line L0 (19, 67.7) -> (21, 67.7)
  line L1 (21, 67.7) -> (21, 108.5)
  line L2 (21, 108.5) -> (19, 108.5)
  line L3 (19, 108.5) -> (19, 67.7)
  line L4 (39, 67.7) -> (41, 67.7)
  line L5 (41, 67.7) -> (41, 108.5)
  line L6 (41, 108.5) -> (39, 108.5)
  line L7 (39, 108.5) -> (39, 67.7)
extrude "Extrude574" add sketch "Sketch580" along normal blind 1.6 from surface at 4.4 separate body makes body 80 at (19.6667, 94.9, 4.4) makes body 81 at (39.6667, 94.9, 4.4)
combine "Combine175" operation add target body 1 tool bodies 80 81
sketch "Sketch581" plane through (0, 0, 0) normal (0, 0, 1) x (1, 0, 0)
  line L0 (41.2, 67.4) -> (65.6, 67.4)
  line L1 (65.6, 67.4) -> (65.6, 98.6)
  line L2 (65.6, 98.6) -> (41.2, 98.6)
  line L3 (41.2, 98.6) -> (41.2, 67.4)
  line L4 (41.2, 98.6) -> (60.4, 98.6)
  line L5 (60.4, 98.6) -> (60.4, 107.9)
  line L6 (60.4, 107.9) -> (41.2, 107.9)
  line L7 (41.2, 107.9) -> (41.2, 98.6)
extrude "Extrude575" cut sketch "Sketch581" along normal blind 11 from surface at -1 bodies 1
sketch "Sketch582" plane through (0, 0, 0) normal (0, 0, 1) x (1, 0, 0)
  line L0 (39.8, 67.4) -> (65.6, 67.4)
  line L1 (65.6, 67.4) -> (65.6, 108.5)
  line L2 (65.6, 108.5) -> (39.8, 108.5)
  line L3 (39.8, 108.5) -> (39.8, 67.4)
extrude "Extrude576" add sketch "Sketch582" along normal blind 4.5 separate body makes body 82
combine "Combine176" operation add target body 1 tool bodies 82
sketch "Sketch583" plane through (0, 0, 0) normal (0, 0, 1) x (1, 0, 0)
  line L0 (39.8, 67.4) -> (42.4, 67.4)
  line L1 (42.4, 67.4) -> (42.4, 108.5)
  line L2 (42.4, 108.5) -> (39.8, 108.5)
  line L3 (39.8, 108.5) -> (39.8, 67.4)
  line L4 (63.4, 67.4) -> (65.6, 67.4)
  line L5 (65.6, 67.4) -> (65.6, 108.5)
  line L6 (65.6, 108.5) -> (63.4, 108.5)
  line L7 (63.4, 108.5) -> (63.4, 67.4)
  line L8 (42.4, 106.5) -> (63.4, 106.5)
  line L9 (63.4, 106.5) -> (63.4, 108.5)
  line L10 (63.4, 108.5) -> (42.4, 108.5)
  line L11 (42.4, 108.5) -> (42.4, 106.5)
extrude "Extrude577" add sketch "Sketch583" along normal blind 3.5 from surface at 4.5 separate body makes body 83
combine "Combine177" operation add target body 1 tool bodies 83
sketch "Sketch584" plane through (0, 0, 0) normal (0, 0, 1) x (1, 0, 0)
  line L0 (20.7, 67.6) -> (39.3, 67.6)
  line L1 (39.3, 67.6) -> (39.3, 107.9)
  line L2 (39.3, 107.9) -> (20.7, 107.9)
  line L3 (20.7, 107.9) -> (20.7, 67.6)
extrude "Extrude578" cut sketch "Sketch584" along normal blind 5.05 from surface at 4.45 bodies 1
sketch "Sketch585" plane through (0, 0, 0) normal (1, 0, 0) x (0, 0, -1)
  line L0 (-13.9219, -5.5) -> (-26.3768, 113)
  line L1 (-26.3768, 113) -> (-40, 113)
  line L2 (-40, 113) -> (-40, -5.5)
  line L3 (-40, -5.5) -> (-13.9219, -5.5)
extrude "Extrude579" cut sketch "Sketch585" along normal mid plane 200 bodies 1
sketch "Sketch586" plane through (0, 0, 0) normal (0, 0, 1) x (1, 0, 0)
  line L0 (0.1, -3.4) -> (84.35, -3.4)
  line L1 (84.35, -3.4) -> (84.35, 110.4)
  line L2 (84.35, 110.4) -> (0.1, 110.4)
  line L3 (0.1, 110.4) -> (0.1, -3.4)
  line L4 (2.5, -1) -> (81.95, -1)
  line L5 (81.95, -1) -> (81.95, 108)
  line L6 (81.95, 108) -> (2.5, 108)
  line L7 (2.5, 108) -> (2.5, -1)
extrude "Extrude580" add sketch "Sketch586" along normal blind 20 from surface at 13.4 separate body makes body 84
sketch "Sketch587" plane through (0, 0, 0) normal (1, 0, 0) x (0, 0, -1)
  line L0 (-16.9219, -5.5) -> (-29.3768, 113)
  line L1 (-29.3768, 113) -> (-40, 113)
  line L2 (-40, 113) -> (-40, -5.5)
  line L3 (-40, -5.5) -> (-16.9219, -5.5)
extrude "Extrude581" cut sketch "Sketch587" along normal mid plane 200 bodies 84
combine "Combine178" operation add target body 1 tool bodies 84
sketch "Sketch588" plane through (0, 0, 0) normal (0, 0, 1) x (1, 0, 0)
  circle A0 centre (20, 102.4) radius 2.1
  circle A1 centre (64, 102.4) radius 2.1
extrude "Extrude582" cut sketch "Sketch588" along normal blind 2.5 bodies 1
sketch "Sketch589" plane through (0, 0, 0) normal (0, 0, 1) x (1, 0, 0)
  circle A0 centre (4.5, 89) radius 2.1
  circle A1 centre (79.95, 89) radius 2.1
extrude "Extrude583" cut sketch "Sketch589" along normal blind 2.5 bodies 1
sketch "Sketch590" plane through (0, 0, 0) normal (0, 0, 1) x (1, 0, 0)
  circle A0 centre (20, 102.4) radius 1.2
  circle A1 centre (64, 102.4) radius 1.2
extrude "Extrude584" cut sketch "Sketch590" along normal blind 18.5627 from surface at 2.3 bodies 1
sketch "Sketch591" plane through (0, 0, 0) normal (0, 0, 1) x (1, 0, 0)
  circle A0 centre (4.5, 89) radius 1.2
  circle A1 centre (79.95, 89) radius 1.2
extrude "Extrude585" cut sketch "Sketch591" along normal blind 17.1543 from surface at 2.3 bodies 1
sketch "Sketch592" plane through (0, 0, 0) normal (0, 0, 1) x (1, 0, 0)
  circle A0 centre (20, 102.4) radius 1.75
  circle A1 centre (64, 102.4) radius 1.75
extrude "Extrude586" cut sketch "Sketch592" along normal blind 5.2 from surface at 20.7627 bodies 1
sketch "Sketch593" plane through (0, 0, 0) normal (0, 0, 1) x (1, 0, 0)
  circle A0 centre (4.5, 89) radius 1.75
  circle A1 centre (79.95, 89) radius 1.75
extrude "Extrude587" cut sketch "Sketch593" along normal blind 5.2 from surface at 19.3543 bodies 1
sketch "Sketch594" plane through (0, 0, 0) normal (0, 0, 1) x (1, 0, 0)
  circle A0 centre (23.175, 0.9) radius 2.1
  circle A1 centre (42.225, 0.9) radius 2.1
  circle A2 centre (61.275, 0.9) radius 2.1
extrude "Extrude588" cut sketch "Sketch594" along normal blind 2.5 bodies 1
sketch "Sketch595" plane through (0, 0, 0) normal (0, 0, 1) x (1, 0, 0)
  circle A0 centre (23.175, 0.9) radius 1.2
  circle A1 centre (42.225, 0.9) radius 1.2
  circle A2 centre (61.275, 0.9) radius 1.2
extrude "Extrude589" cut sketch "Sketch595" along normal blind 7.8946 from surface at 2.3 bodies 1
sketch "Sketch596" plane through (0, 0, 0) normal (0, 0, 1) x (1, 0, 0)
  circle A0 centre (23.175, 0.9) radius 1.75
  circle A1 centre (42.225, 0.9) radius 1.75
  circle A2 centre (61.275, 0.9) radius 1.75
extrude "Extrude590" cut sketch "Sketch596" along normal blind 5.2 from surface at 10.0946 bodies 1
sketch "Sketch597" plane through (0, 0, 0) normal (0, 0, 1) x (1, 0, 0)
  line L0 (25.5, 107) -> (34.5, 107)
  line L1 (34.5, 107) -> (34.5, 113.5)
  line L2 (34.5, 113.5) -> (25.5, 113.5)
  line L3 (25.5, 113.5) -> (25.5, 107)
extrude "Extrude591" cut sketch "Sketch597" along normal blind 4 from surface at 4.5 bodies 1
sketch "Sketch598" plane through (0, 0, 0) normal (0, 0, 1) x (1, 0, 0)
  line L0 (-1, 36.05) -> (3.5, 36.05)
  line L1 (3.5, 36.05) -> (3.5, 44.95)
  line L2 (3.5, 44.95) -> (-1, 44.95)
  line L3 (-1, 44.95) -> (-1, 36.05)
extrude "Extrude592" cut sketch "Sketch598" along normal blind 4.2 from surface at 6 bodies 1
sketch "Sketch599" plane through (0, 0, 0) normal (1, 0, 0) x (0, 0, -1)
  circle A0 centre (-7.5, 75) radius 1.25
extrude "Extrude593" cut sketch "Sketch599" along normal blind 4.5 from surface at 81 bodies 1
sketch "Sketch600" plane through (0, 0, 0) normal (0, 0, 1) x (1, 0, 0)
  line L0 (2.725, -0.78) -> (81.725, -0.78)
  line L1 (81.725, -0.78) -> (81.725, 107.75)
  line L2 (81.725, 107.75) -> (2.725, 107.75)
  line L3 (2.725, 107.75) -> (2.725, -0.78)
extrude "Extrude594" add sketch "Sketch600" along normal blind 2.5 separate body makes body 85
sketch "Sketch601" plane through (0, 0, 0) normal (0, 0, 1) x (1, 0, 0)
  line L0 (6.65, 6.63) -> (20.65, 6.63)
  line L1 (20.65, 6.63) -> (20.65, 20.63)
  line L2 (20.65, 20.63) -> (6.65, 20.63)
  line L3 (6.65, 20.63) -> (6.65, 6.63)
  line L4 (6.65, 25.68) -> (20.65, 25.68)
  line L5 (20.65, 25.68) -> (20.65, 39.68)
  line L6 (20.65, 39.68) -> (6.65, 39.68)
  line L7 (6.65, 39.68) -> (6.65, 25.68)
  line L8 (6.65, 44.73) -> (20.65, 44.73)
  line L9 (20.65, 44.73) -> (20.65, 58.73)
  line L10 (20.65, 58.73) -> (6.65, 58.73)
  line L11 (6.65, 58.73) -> (6.65, 44.73)
  line L12 (6.65, 63.78) -> (20.65, 63.78)
  line L13 (20.65, 63.78) -> (20.65, 77.78)
  line L14 (20.65, 77.78) -> (6.65, 77.78)
  line L15 (6.65, 77.78) -> (6.65, 63.78)
  line L16 (25.7, 6.63) -> (39.7, 6.63)
  line L17 (39.7, 6.63) -> (39.7, 20.63)
  line L18 (39.7, 20.63) -> (25.7, 20.63)
  line L19 (25.7, 20.63) -> (25.7, 6.63)
  line L20 (25.7, 25.68) -> (39.7, 25.68)
  line L21 (39.7, 25.68) -> (39.7, 39.68)
  line L22 (39.7, 39.68) -> (25.7, 39.68)
  line L23 (25.7, 39.68) -> (25.7, 25.68)
  line L24 (25.7, 44.73) -> (39.7, 44.73)
  line L25 (39.7, 44.73) -> (39.7, 58.73)
  line L26 (39.7, 58.73) -> (25.7, 58.73)
  line L27 (25.7, 58.73) -> (25.7, 44.73)
  line L28 (25.7, 63.78) -> (39.7, 63.78)
  line L29 (39.7, 63.78) -> (39.7, 77.78)
  line L30 (39.7, 77.78) -> (25.7, 77.78)
  line L31 (25.7, 77.78) -> (25.7, 63.78)
  line L32 (44.75, 6.63) -> (58.75, 6.63)
  line L33 (58.75, 6.63) -> (58.75, 20.63)
  line L34 (58.75, 20.63) -> (44.75, 20.63)
  line L35 (44.75, 20.63) -> (44.75, 6.63)
  line L36 (44.75, 25.68) -> (58.75, 25.68)
  line L37 (58.75, 25.68) -> (58.75, 39.68)
  line L38 (58.75, 39.68) -> (44.75, 39.68)
  line L39 (44.75, 39.68) -> (44.75, 25.68)
  line L40 (44.75, 44.73) -> (58.75, 44.73)
  line L41 (58.75, 44.73) -> (58.75, 58.73)
  line L42 (58.75, 58.73) -> (44.75, 58.73)
  line L43 (44.75, 58.73) -> (44.75, 44.73)
  line L44 (44.75, 63.78) -> (58.75, 63.78)
  line L45 (58.75, 63.78) -> (58.75, 77.78)
  line L46 (58.75, 77.78) -> (44.75, 77.78)
  line L47 (44.75, 77.78) -> (44.75, 63.78)
  line L48 (63.8, 6.63) -> (77.8, 6.63)
  line L49 (77.8, 6.63) -> (77.8, 20.63)
  line L50 (77.8, 20.63) -> (63.8, 20.63)
  line L51 (63.8, 20.63) -> (63.8, 6.63)
  line L52 (63.8, 25.68) -> (77.8, 25.68)
  line L53 (77.8, 25.68) -> (77.8, 39.68)
  line L54 (77.8, 39.68) -> (63.8, 39.68)
  line L55 (63.8, 39.68) -> (63.8, 25.68)
  line L56 (63.8, 44.73) -> (77.8, 44.73)
  line L57 (77.8, 44.73) -> (77.8, 58.73)
  line L58 (77.8, 58.73) -> (63.8, 58.73)
  line L59 (63.8, 58.73) -> (63.8, 44.73)
  line L60 (63.8, 63.78) -> (77.8, 63.78)
  line L61 (77.8, 63.78) -> (77.8, 77.78)
  line L62 (77.8, 77.78) -> (63.8, 77.78)
  line L63 (63.8, 77.78) -> (63.8, 63.78)
  circle A0 centre (20, 102.964) radius 1.2
  circle A1 centre (64, 102.964) radius 1.2
  circle A2 centre (4.5, 89.4902) radius 1.2
  circle A3 centre (79.95, 89.4902) radius 1.2
  circle A4 centre (23.175, 0.905) radius 1.2
  circle A5 centre (42.225, 0.905) radius 1.2
  circle A6 centre (61.275, 0.905) radius 1.2
  circle A7 centre (13.65, 89.83) radius 3.6
  circle A8 centre (70.8, 89.83) radius 3.6
  line L64 (29.725, 83.83) -> (54.725, 83.83)
  line L65 (54.725, 83.83) -> (54.725, 101.33)
  line L66 (54.725, 101.33) -> (29.725, 101.33)
  line L67 (29.725, 101.33) -> (29.725, 83.83)
  line L68 (2.725, 1.22) -> (2.725, -0.78)
  line L69 (2.725, -0.78) -> (4.725, -0.78)
  arc A9 (2.725, 1.22) -> (4.725, -0.78) centre (4.725, 1.22) ccw
  line L70 (79.725, -0.78) -> (81.725, -0.78)
  line L71 (81.725, -0.78) -> (81.725, 1.22)
  arc A10 (79.725, -0.78) -> (81.725, 1.22) centre (79.725, 1.22) ccw
  line L72 (2.725, 105.75) -> (2.725, 107.75)
  line L73 (2.725, 107.75) -> (4.725, 107.75)
  arc A11 (4.725, 107.75) -> (2.725, 105.75) centre (4.725, 105.75) ccw
  line L74 (81.725, 105.75) -> (81.725, 107.75)
  line L75 (81.725, 107.75) -> (79.725, 107.75)
  arc A12 (81.725, 105.75) -> (79.725, 107.75) centre (79.725, 105.75) ccw
extrude "Extrude595" cut sketch "Sketch601" along normal blind 3 from surface at -0.5 bodies 85
sketch "Sketch602" plane through (0, 0, 0) normal (0, 0, 1) x (1, 0, 0)
  line L0 (26.725, 79.83) -> (57.725, 79.83)
  line L1 (57.725, 79.83) -> (57.725, 83.83)
  line L2 (57.725, 83.83) -> (26.725, 83.83)
  line L3 (26.725, 83.83) -> (26.725, 79.83)
  line L4 (26.725, 101.33) -> (57.725, 101.33)
  line L5 (57.725, 101.33) -> (57.725, 105.33)
  line L6 (57.725, 105.33) -> (26.725, 105.33)
  line L7 (26.725, 105.33) -> (26.725, 101.33)
extrude "Extrude596" cut sketch "Sketch602" along normal blind 1.5 from surface at -0.5 bodies 85